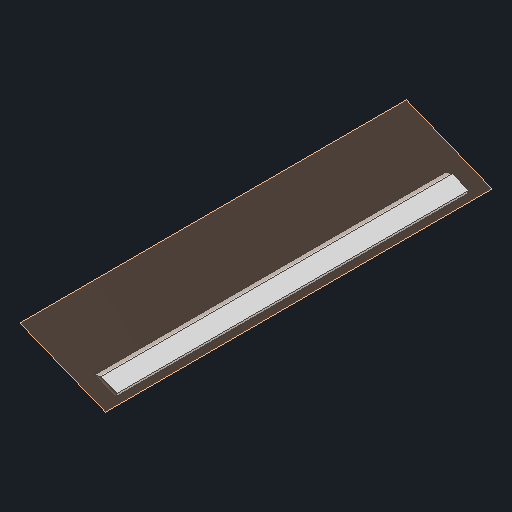
# Autodesk Inventor part: platte
Saved by Autodesk Inventor 2023 (Build 270158000, 158)
## iProperties
Created: 2022-06-24
Part Number: platte
Material: Generic
Document SubType Name: Modeling
Designer: bananenbrot
Density: 1 g/cm^3
Appearance: Default
Author: bananenbrot
Autodesk Inventor part; units mm, degrees
ref_plane "YZ Plane" through (0, 0, 0) normal (1, 0, 0) x (0, 1, 0)
ref_plane "XZ Plane" through (0, 0, 0) normal (0, 1, 0) x (-1, 0, 0)
ref_plane "Work Plane1" through (0, 0, 0) normal (0, 0, 1) x (1, 0, 0)
sketch "Sketch1" plane through (0, 0, 0) normal (0, 0, 1) x (1, 0, 0)
  arc A0 (11.7519, -6.4859) -> (17.0448, -5.0515) centre (7.6561, 19.1093) ccw projected
  line L0 (29.0445, -13.4142) -> (11.7519, -6.4859) projected
  arc A1 (11.7519, -6.4859) -> (17.0448, -5.0515) centre (7.6561, 19.1093) ccw projected
  line L1 (29.0445, -13.4142) -> (11.7519, -6.4859) projected
  line L2 (17.0448, -5.0515) -> (-15.8175, 8.1147)
  line L3 (11.7519, -6.4859) -> (-12.9792, 3.4226)
  line L4 (30.2718, -10.3509) -> (29.0445, -13.4142) projected
  line L5 (17.0448, -5.0515) -> (30.2718, -10.3509) projected
  line L6 (30.2718, -10.3509) -> (29.0445, -13.4142) projected
  line L7 (17.0448, -5.0515) -> (30.2718, -10.3509) projected
  point P0 (0, 0)
  constraints: 4 end point, 1 collinear
extrude "Extrusion1" add sketch "Sketch1" along normal blind 288
sketch "Sketch2" plane through (-30.2513, 13.8976, 288) normal (0.3719, 0.9283, 0) x (0.9283, -0.3719, 0)
  circle A0 centre (7.1485, 7.8489) radius 2
  point P0 (33.25, 288)
  dimension "d2" = 4
  constraints: 1 centre point
  measures "d2" diameter of A0
extrude "Extrusion2" [suppressed]
pattern_linear "Rectangular Pattern1" [suppressed]
ref_plane "Work Plane2" through (-30.8649, 12.366, 288) normal (0.3719, 0.9283, 0) x (0.9283, -0.3719, 0)
body "Solid1"
